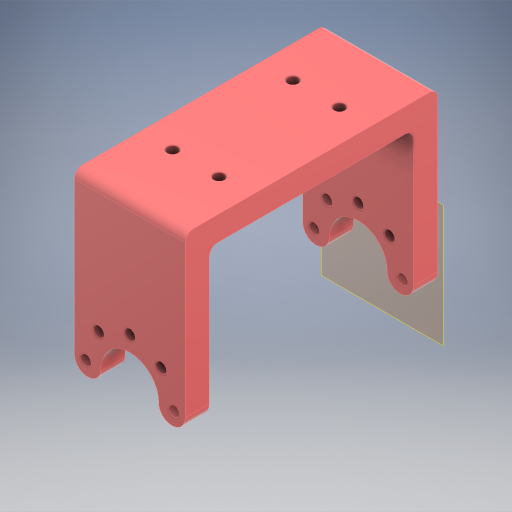
# Autodesk Inventor part: foot_right_64
Saved by Autodesk Inventor 2024 (Build 280153000, 153)
## iProperties
Created: 2024-09-04
Part Number: foot_right_64
Material: PMMA 플라스틱
Document SubType Name: Modeling
Designer: msi
Density: 1.188 g/cm^3
Appearance: 매끄러움 - 빨간색
Author: msi
Autodesk Inventor part; units mm, degrees
ref_plane "YZ Plane" through (0, 0, 0) normal (1, 0, 0) x (0, 1, 0)
ref_plane "XZ Plane" through (0, 0, 0) normal (0, 1, 0) x (-1, 0, 0)
ref_plane "XY Plane" through (0, 0, 0) normal (0, 0, 1) x (1, 0, 0)
ref_plane "작업 평면1" through (0, 0, 0) normal (0, 0, 1) x (1, 0, 0)
sketch "스케치1" plane through (0, 0, 0) normal (0, 0, 1) x (1, 0, 0)
  circle A0 centre (0, 0) radius 13.8 projected
  circle A1 centre (0, 0) radius 7.2 projected
  circle A2 centre (0, -11) radius 1.2813 projected
  circle A3 centre (-7.7782, -7.7782) radius 1.2813 projected
  circle A4 centre (-11, 0) radius 1.2813 projected
  circle A5 centre (-7.7782, 7.7782) radius 1.2813 projected
  circle A6 centre (0, 11) radius 1.2813 projected
  circle A7 centre (7.7782, 7.7782) radius 1.2813 projected
  circle A8 centre (11, 0) radius 1.2813 projected
  circle A9 centre (7.7782, -7.7782) radius 1.2813 projected
  line L0 (-13.8, 0) -> (-13.8, 13.8)
  line L1 (-13.8, 13.8) -> (13.8, 13.8)
  line L2 (13.8, 13.8) -> (13.8, 0)
  circle A10 centre (0, 0) radius 7.25
  arc A11 (7.2344, 0.4753) -> (13.8, 0) centre (10.5, 0) ccw
  arc A12 (-13.8, 0) -> (-7.2344, 0.4753) centre (-10.5, 0) ccw
  line L3 (7.25, 0) -> (7.2, 0)
  line L4 (-7.2, 0) -> (-7.25, 0)
  circle A13 centre (11, 0) radius 1.35
  circle A14 centre (7.7782, 7.7782) radius 1.35
  circle A15 centre (0, 11) radius 1.35
  circle A16 centre (-7.7782, 7.7782) radius 1.35
  circle A17 centre (-11, 0) radius 1.35
  line L5 (13.8, 13.8) -> (-13.8, 13.8)
  line L6 (-13.8, 13.8) -> (-13.8, 33.8)
  line L7 (-13.8, 33.8) -> (13.8, 33.8)
  line L8 (13.8, 33.8) -> (13.8, 13.8)
  line L9 (3, 33.8) -> (-3, 33.8)
  line L10 (-3, 33.8) -> (-3, 39.8)
  line L11 (-3, 39.8) -> (3, 39.8)
  line L12 (3, 39.8) -> (3, 33.8)
  point P0 (0, 0)
  point P1 (-7.2344, -0.4753)
  point P2 (7.2344, -0.4753)
  dimension "d0" = 14.5
  dimension "d1" = 2.7
  dimension "d2" = 2.7
  dimension "d3" = 2.7
  dimension "d4" = 2.7
  dimension "d5" = 2.7
  dimension "d6" = 20
  dimension "d7" = 6
  dimension "d8" = 6
  constraints: 26 end point, 11 point on circle, 8 centre point, 7 parallel, 6 coincident, 4 horizontal, 4 perpendicular, 1 horizontal alignment, 1 point on line, 1 other
  measures "d0" diameter of A10
  measures "d1" diameter of A13
  measures "d2" diameter of A14
  measures "d3" diameter of A15
  measures "d4" diameter of A16
  measures "d5" diameter of A17
  measures "d6" distance of L5.end L6.end
  measures "d7" distance of L10.end L11.end
  measures "d8" distance of L9.end L10.end
extrude "돌출1" add sketch "스케치1" along normal blind 6 contours L0 L1 A0 | A0 A11 A10 A12 | A0 L1 L2 | L1 L6 L7 L8 | L10 L11 L12 L7 picked at (-4.6271, 10.5053)
sketch "스케치2" plane through (-3, 39.8, 0) normal (0, 1, 0) x (1, 0, 0)
  circle A0 centre (-5, -3) radius 1.35
  circle A1 centre (11, -3) radius 1.35
  point P0 (3, 0)
  dimension "d11" = 2.7
  dimension "d12" = 2.7
  constraints: 2 centre point
  measures "d11" diameter of A0
  measures "d12" diameter of A1
extrude "돌출2" cut sketch "스케치2" against normal blind 20
sketch "스케치3" plane through (0, 0, 6) normal (0, 0, 1) x (1, 0, 0)
  line L0 (-9.35, 33.8) -> (-9.35, 19.8) projected
  line L1 (-6.65, 33.8) -> (-6.65, 19.8) projected
  line L2 (15, 15) -> (-15, 15) projected
  line L3 (6.65, 33.8) -> (6.65, 19.8) projected
  line L4 (9.35, 33.8) -> (9.35, 19.8) projected
  line L5 (9.35, 26.8) -> (6.65, 26.8)
  line L6 (-6.65, 26.8) -> (-9.35, 26.8)
  line L7 (10.6, 27.9) -> (5.4, 27.9)
  line L8 (5.4, 27.9) -> (5.4, 25.7)
  line L9 (5.4, 25.7) -> (10.6, 25.7)
  line L10 (10.6, 25.7) -> (10.6, 27.9)
  line L11 (10.6, 27.9) -> (5.4, 25.7) construction
  line L12 (5.4, 27.9) -> (10.6, 25.7) construction
  line L13 (-5.4, 27.9) -> (-10.6, 27.9)
  line L14 (-10.6, 27.9) -> (-10.6, 25.7)
  line L15 (-10.6, 25.7) -> (-5.4, 25.7)
  line L16 (-5.4, 25.7) -> (-5.4, 27.9)
  line L17 (-5.4, 27.9) -> (-10.6, 25.7) construction
  line L18 (-10.6, 27.9) -> (-5.4, 25.7) construction
  point P0 (0, 0)
  point P1 (8, 26.8)
  point P2 (-8, 26.8)
  dimension "d15" = 5.2
  dimension "d16" = 2.2
  dimension "d17" = 5.2
  dimension "d18" = 2.2
  constraints: 28 end point, 10 midpoint, 4 parallel, 2 horizontal, 2 perpendicular
  measures "d15" distance of L9.end L8.end
  measures "d16" distance of L8.end L7.end
  measures "d17" distance of L15.end L14.end
  measures "d18" distance of L14.end L13.end
extrude "돌출3" cut sketch "스케치3" against normal blind 20
sketch "스케치4" plane through (-3, 39.8, 0) normal (0, 1, 0) x (1, 0, 0)
  line L0 (-2, 0) -> (8, 0)
  line L1 (8, 0) -> (8, -6)
  line L2 (8, -6) -> (-2, -6)
  line L3 (-2, -6) -> (-2, 0)
  line L4 (-2, 0) -> (8, -6) construction
  line L5 (8, 0) -> (-2, -6) construction
  point P0 (3, 0)
  point P1 (3, -3)
  dimension "d21" = 10
  dimension "d22" = 6
  constraints: 12 end point, 2 midpoint, 2 parallel, 1 horizontal, 1 perpendicular
  measures "d21" distance of L1.end L2.end
  measures "d22" distance of L0.end L1.end
extrude "돌출4" add sketch "스케치4" against normal blind 6
sketch "스케치5" plane through (0, 0, 6) normal (0, 0, 1) x (1, 0, 0)
  line L0 (-5, 33.8) -> (-13.8, 33.8) projected
  line L1 (13.8, 33.8) -> (5, 33.8) projected
  line L2 (-5, 39.8) -> (-5, 33.8) projected
  line L3 (-13.8, 33.8) -> (-13.8, 0) projected
  line L4 (13.8, 0) -> (13.8, 33.8) projected
  line L5 (-5, 39.8) -> (5, 39.8) projected
  line L6 (-13.8, 33.8) -> (13.8, 33.8)
  line L7 (13.8, 33.8) -> (13.8, 39.8)
  line L8 (13.8, 39.8) -> (-13.8, 39.8)
  line L9 (-13.8, 39.8) -> (-13.8, 33.8)
  point P0 (0, 0)
  point P1 (5, 39.8)
  constraints: 8 end point, 2 parallel, 1 horizontal, 1 perpendicular
extrude "돌출5" cut sketch "스케치5" against normal blind 10
sketch "스케치6" plane through (0, 0, 6) normal (0, 0, 1) x (1, 0, 0)
  line L0 (-13.8, 33.8) -> (-13.8, 0) projected
  line L1 (13.8, 33.8) -> (-13.8, 33.8) projected
  line L2 (13.8, 0) -> (13.8, 33.8) projected
  line L3 (-13.8, 33.8) -> (13.8, 33.8)
  line L4 (13.8, 33.8) -> (13.8, 14.8)
  line L5 (13.8, 14.8) -> (-13.8, 14.8)
  line L6 (-13.8, 14.8) -> (-13.8, 33.8)
  point P0 (0, 0)
  point P1 (-13.8, 14.8)
  dimension "d27" = 19
  constraints: 8 end point, 2 parallel, 1 horizontal, 1 perpendicular, 1 point on line
  measures "d27" distance of L3.end L4.end
extrude "돌출6" add sketch "스케치6" against normal blind 6
sketch "스케치7" plane through (0, 0, 6) normal (0, 0, 1) x (1, 0, 0)
  line L0 (13.8, 33.8) -> (-13.8, 33.8) projected
  line L1 (-13.8, 33.8) -> (-13.8, 0) projected
  arc A0 (-13.8, 0) -> (-7.2344, -0.4753) centre (-10.5, 0) ccw projected
  line L2 (13.8, 0) -> (13.8, 33.8) projected
  line L3 (-13.8, 33.8) -> (13.8, 33.8)
  line L4 (13.8, 33.8) -> (13.8, 39.8)
  line L5 (13.8, 39.8) -> (-13.8, 39.8)
  line L6 (-13.8, 39.8) -> (-13.8, 33.8)
  point P0 (0, 0)
  dimension "d30" = 6
  constraints: 8 end point, 2 parallel, 1 horizontal, 1 perpendicular
  measures "d30" distance of L4.end L3.end
extrude "돌출7" add sketch "스케치7" along normal blind 25.45
sketch "스케치8" plane through (0, 0, 6) normal (0, 0, -1) x (-1, 0, 0)
  line L0 (13.8, 39.8) -> (13.8, 33.8) projected
  line L1 (-13.8, 33.8) -> (13.8, 33.8) projected
  line L2 (13.8, 39.8) -> (13.8, 33.8) projected
  line L3 (-13.8, 39.8) -> (13.8, 39.8) projected
  line L4 (-13.8, 33.8) -> (-13.8, 39.8) projected
  line L5 (-13.8, 39.8) -> (13.8, 39.8) projected
  line L6 (-13.8, 39.8) -> (13.8, 39.8)
  line L7 (13.8, 39.8) -> (13.8, 33.8)
  line L8 (13.8, 33.8) -> (-13.8, 33.8)
  line L9 (-13.8, 33.8) -> (-13.8, 39.8)
  point P0 (0, 0)
  constraints: 8 end point, 2 parallel, 1 horizontal, 1 perpendicular
extrude "돌출8" add sketch "스케치8" along normal blind 6
sketch "스케치9" plane through (-13.8, 39.8, 31.45) normal (0, 1, 0) x (1, 0, 0)
  line L0 (0, 31.45) -> (0, 0) projected
  line L1 (27.6, 0) -> (0, 0) projected
  line L2 (27.6, 31.45) -> (27.6, 0) projected
  line L3 (0, 31.45) -> (27.6, 31.45) projected
  line L4 (27.6, 25.45) -> (0, 25.45) projected
  circle A0 centre (8, 15) radius 1.35
  circle A1 centre (19.6, 15) radius 1.35
  point P0 (13.8, 31.45)
  dimension "d35" = 2.7
  dimension "d36" = 2.7
  constraints: 2 centre point
  measures "d35" diameter of A0
  measures "d36" diameter of A1
extrude "돌출9" cut sketch "스케치9" against normal blind 6 contours A0 | A1
fillet "모깎기1" radius 2 2 edges at (0, 39.8, 0) (0, 33.8, 6)
mirror "미러1" about plane through (0, 36.8, 31.45) normal (0, 0, 1)
